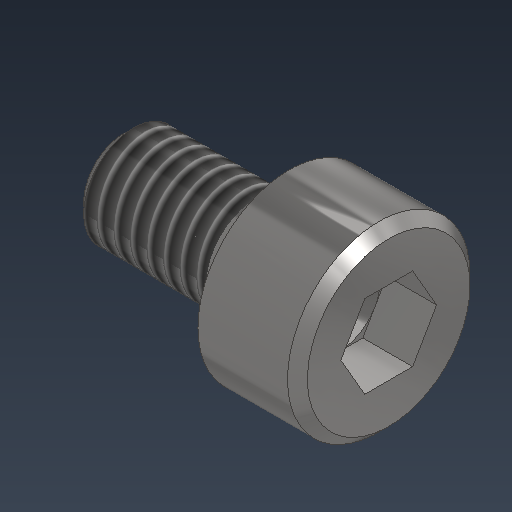
# Autodesk Inventor part: CB3-5
Saved by Autodesk Inventor 2021 (Build 250183000, 183)
## iProperties
Category: PARTsolutions
Company: MISUMI
Part Number: CB3-5
Material: 鋼、炭素鋼
Catalog Web Link: www.cadenas.de
Description: 在庫有
Vendor: MISUMI
Document SubType Name: Modeling
Designer: partserver
Manufacturer: MISUMI
Mass: 0.759793 g
Surface Area: 1.54672 cm^2
Volume: 0.096789 cm^3
Density: 7.85 g/cm^3
Appearance: 半つや出し
PSOL_IDENT_0: {$CADENAS_DATA\23d-libs\misumi\metric\27_screws_nuts\cb_fa.prj},148 {VTYP=3D},{NB=CB3-5},{LINA=CB3-5
PSOL_IDENT_1: },{NN=CB},{DATE=09.09.2019 15:27:56},{GEOMDATE=17.02.2014 00:00:00},{VERSION=},{LINEID=60},{WBVAR=L}
PSOL_IDENT_2: ,{WBNUMERIC=L}  {NB=CB3-5},{LINA=CB3-5},{KT=DUMMY},{PN=CB3-5},{MAT=4137 Steel},{HARD=38~43HRC},{ST=B
PSOL_IDENT_3: lack Oxide},{M=3},{L=5},{LL=Full Thread},{L1=18},{TYPE=CB},{M1=3.000},{L0=5,6,8,10,12,14,15,16,18,20
PSOL_IDENT_4: ,22,25,30,35,40,45,50,55},{NDM=3},{KDM=2.385665},{MP=3x0.5},{P=0.5},{A=5.5},{E=3.0},{B=2.5},{V=0.3}
NB: CB3-5
NN: CB
NT: Hexagon Socket Head Cap Screws
NBSYN: $PN.
LINA: CB3-5
CATALOG: Misumi
PN: CB3-5
MAT: 4137 Steel
HARD: 38~43HRC
ST: Black Oxide
M: 3
L: 5
LL: Full Thread
MP: 3x0.5
A: 5.5
E: 3
B: 2.5
SUPPLIER: MISUMI
ARTICLENO: CB3-5
BOMINFO: CB3-5
CREATOR: CADENAS GmbH
d12: 0.000 mm
d13: 0.000 mm
購入先: ミスミ
在庫数: 56.0
Title: CB3-5
Author: Cadenas PARTsolutions
Comments: Hexagon Socket Head Cap Screws
Autodesk Inventor part; units mm, degrees
sketch "Sketch_1" plane through (0, 0, 0) normal (0, 0, 1) x (1, 0, 0)
  line L0 (5, 0) -> (-3, 0)
  line L1 (-3, 0) -> (-3, 2.45)
  line L2 (-3, 2.45) -> (-2.7, 2.75)
  line L3 (-2.7, 2.75) -> (0, 2.75)
  line L4 (0, 2.75) -> (0, 1.5)
  line L5 (0, 1.5) -> (4.6935, 1.5)
  line L6 (4.6935, 1.5) -> (5, 1.1935)
  line L7 (5, 1.1935) -> (5, 0)
  line L8 (5, 0) -> (-3, 0)
  constraints: 18 end point
revolve "Revolution1" add sketch "Sketch_1" angle 360 about axis through (5, 0, 0) along (1, 0, 0)
thread "Thread1" size "M3x0.5" class "6g" standard "ISO Metric profile" length 3.6935
sketch "Sketch2" plane through (-3, 0, 0) normal (-1, 0, 0) x (0, 0, 1)
  point P0 (0, 0)
hole "Hole1" at (-3, 0, 0) direction (1, 0, 0) diameter 2.5 depth 1.5 tip angle 150
sketch "Sketch_3" plane through (-3, 0, 0) normal (1, 0, 0) x (0, 0, -1)
  line L0 (-1.25, -0.7217) -> (0, -1.4434)
  line L1 (0, -1.4434) -> (1.25, -0.7217)
  line L2 (1.25, -0.7217) -> (1.25, 0.7217)
  line L3 (1.25, 0.7217) -> (0, 1.4434)
  line L4 (0, 1.4434) -> (-1.25, 0.7217)
  line L5 (-1.25, 0.7217) -> (-1.25, -0.7217)
  constraints: 12 end point
extrude "Extrusion1" cut sketch "Sketch_3" along normal blind 1.5
ref_plane "bolt_to_nut_XY" through (5, 0, 0) normal (1, 0, 0) x (0, 0, -1)
ref_plane "bolt_to_nut_YZ" through (5, 0, 0) normal (0, 0, -1) x (0, 1, 0)
ref_plane "bolt_to_nut_ZX" through (5, 0, 0) normal (0, 1, 0) x (1, 0, 0)
ref_plane "screw1_XY" through (0, 0, 0) normal (1, 0, 0) x (0, 0, -1)
ref_plane "screw1_YZ" through (0, 0, 0) normal (0, 0, -1) x (0, 1, 0)
ref_plane "screw1_ZX" through (0, 0, 0) normal (0, 1, 0) x (1, 0, 0)
body "Solid1"
